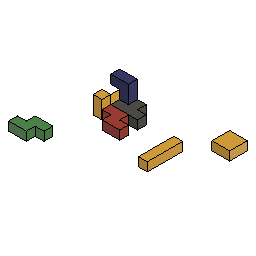
Day1 - Tetris v1 (Autodesk Fusion 360 design; units mm, degrees)
Autodesk Fusion 360 part; units mm, degrees
sketch "Sketch1" plane through (0, 0, 0) normal (0, 0, 1) x (1, 0, 0)
  line L0 (18.2499, 6.5974) -> (48.2499, 6.5974)
  line L1 (48.2499, 6.5974) -> (48.2499, 16.5974)
  line L2 (48.2499, 16.5974) -> (38.2499, 16.5974)
  line L3 (38.2499, 16.5974) -> (38.2499, 26.5974)
  line L4 (38.2499, 26.5974) -> (28.2499, 26.5974)
  line L5 (28.2499, 26.5974) -> (28.2499, 16.4444)
  line L6 (28.2499, 16.4444) -> (18.2499, 16.4444)
  line L7 (18.2499, 16.4444) -> (18.2499, 6.5974)
  line L8 (64.0982, 5.113) -> (74.0982, 5.113)
  line L9 (74.0982, 5.113) -> (74.0982, 45.113)
  line L10 (74.0982, 45.113) -> (64.0982, 45.113)
  line L11 (64.0982, 45.113) -> (64.0982, 5.113)
  line L12 (14.3073, -13.3358) -> (14.3073, -23.3358)
  line L13 (14.3073, -23.3358) -> (24.3073, -23.3358)
  line L14 (24.3073, -23.3358) -> (24.3073, -33.3358)
  line L15 (24.3073, -33.3358) -> (44.3073, -33.3358)
  line L16 (44.3073, -33.3358) -> (44.3073, -23.3358)
  line L17 (44.3073, -23.3358) -> (34.3073, -23.3358)
  line L18 (34.3073, -23.3358) -> (34.3073, -13.3358)
  line L19 (34.3073, -13.3358) -> (14.3073, -13.3358)
  line L20 (0, 0) -> (0, -43.8232) construction
  line L21 (-24.3073, -33.3358) -> (-44.3073, -33.3358)
  line L22 (-14.3073, -23.3358) -> (-24.3073, -23.3358)
  line L23 (-14.3073, -13.3358) -> (-14.3073, -23.3358)
  line L24 (-24.3073, -23.3358) -> (-24.3073, -33.3358)
  line L25 (-44.3073, -33.3358) -> (-44.3073, -23.3358)
  line L26 (-34.3073, -13.3358) -> (-14.3073, -13.3358)
  line L27 (-34.3073, -23.3358) -> (-34.3073, -13.3358)
  line L28 (-44.3073, -23.3358) -> (-34.3073, -23.3358)
  line L29 (15.2563, 69.8959) -> (15.2563, 49.8959)
  line L30 (15.2563, 49.8959) -> (5.2563, 49.8959)
  line L31 (5.2563, 49.8959) -> (5.2563, 39.8959)
  line L32 (5.2563, 39.8959) -> (25.2563, 39.8959)
  line L33 (25.2563, 39.8959) -> (25.2563, 69.8959)
  line L34 (25.2563, 69.8959) -> (15.2563, 69.8959)
  line L35 (-25.2563, 69.8959) -> (-15.2563, 69.8959)
  line L36 (-25.2563, 39.8959) -> (-25.2563, 69.8959)
  line L37 (-5.2563, 39.8959) -> (-25.2563, 39.8959)
  line L38 (-15.2563, 69.8959) -> (-15.2563, 49.8959)
  line L39 (-5.2563, 49.8959) -> (-5.2563, 39.8959)
  line L40 (-15.2563, 49.8959) -> (-5.2563, 49.8959)
  line L41 (110.0191, 62.3742) -> (90.0191, 62.3742)
  line L42 (90.0191, 62.3742) -> (90.0191, 82.3742)
  line L43 (90.0191, 82.3742) -> (110.0191, 82.3742)
  line L44 (110.0191, 82.3742) -> (110.0191, 62.3742)
  line L45 (110.0191, 62.3742) -> (90.0191, 82.3742) construction
  line L46 (90.0191, 62.3742) -> (110.0191, 82.3742) construction
  dimension "d2" = 10
  dimension "d3" = 10
  dimension "d4" = 40
  dimension "d5" = 20
  dimension "d6" = 10
  dimension "d7" = 30
  dimension "d8" = 10
  dimension "d9" = 20
  measures "d4" distance of L20.start
  measures "d8" distance of L20.start
extrude "Extrude1" add sketch "Sketch1" along normal blind 10 makes body 1 at (31.5832, 9.8797, 0) makes body 2 at (-21.923, 53.2292, 0) makes body 3 at (64.0982, 31.7797, 3.3333) makes body 4 at (-34.3073, -30.0024, 0) makes body 5 at (21.923, 53.2292, 0) makes body 6 at (103.3524, 69.0408, 0) makes body 7 at (34.3073, -30.0024, 0)
copy_body "Body->Comp1" bodies 1 removing the originals makes body 8 in component "Component"
copy_body "Body->Comp2" bodies 2 removing the originals makes body 9 in component "Component'"
copy_body "Body->Comp3" bodies 3 removing the originals makes body 10 in component "Component''"
copy_body "Body->Comp4" bodies 7 removing the originals makes body 11 in component "Component'''"
copy_body "Body->Comp5" bodies 4 removing the originals makes body 12 in component "Component''''"
copy_body "Body->Comp6" bodies 5 removing the originals makes body 13 in component "Component'''''"
copy_body "Body->Comp7" bodies 6 removing the originals makes body 14 in component "Component''''''"
component "Component" placed x (1, 0, 0) y (0, 1, 0) z (0, 0, 1) at (-22.9936, 36.2293, -2.2222)
component "Component'" placed x (0, 0, 1) y (0, 1, 0) z (-1, 0, 0) at (-4.7437, -7.2222, 23.0341)
component "Component''" placed x (1, 0, 0) y (0, 1, 0) z (0, 0, 1) at (0, 0, 0)
component "Component'''" placed x (1, 0, 0) y (0, 1, 0) z (0, 0, 1) at (-19.051, 56.1625, -2.2222)
component "Component''''" placed x (1, 0, 0) y (0, 1, 0) z (0, 0, 1) at (0, 0, 0)
component "Component'''''" placed x (1, 0, 0) y (0, 0, -1) z (0, 1, 0) at (-20, 52.6737, 67.6737)
component "Component''''''" placed x (1, 0, 0) y (0, 1, 0) z (0, 0, 1) at (0, 0, 0)
equation "b = 10 mm"
equation "d2 = b"
equation "d3 = b"
equation "d4 = b * 4"
equation "d5 = b * 2"
equation "d6 = b"
equation "d7 = b * 3"
equation "d8 = b"
equation "d9 = b * 2"
equation "d10 = b"
